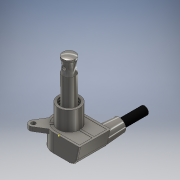
# Autodesk Inventor part: Peça 7
Saved by Autodesk Inventor 2016 (Build 200138000, 138)
## iProperties
Created: 2018-12-04
Part Number: Peça 7
Material: Generic
Document SubType Name: Sheet Metal
Designer: dqm_r
Density: 1 g/cm^3
Sheet Metal Rule: Default_mm
Appearance: Black
Author: dqm_r
Autodesk Inventor part; units mm, degrees
sketch "Sketch2" plane through (0, 0, 0) normal (0, 1, 0) x (-1, 0, 0)
  line L0 (10, 0) -> (-10, 0)
  line L1 (10, 0) -> (10, -9)
  line L2 (10, -9) -> (-5, -9)
  line L3 (-8.769781, -5.931826) -> (-10, 0)
  arc A0 (-8.769781, -5.931826) -> (-5, -9) centre (-5, -5.15) ccw
  line L4 (-10, 0) -> (-5, 0)
  point P0 (0, 0)
  point P1 (0, 0)
  dimension "d3" = 20
  dimension "d4" = 9
  dimension "d5" = 15
  dimension "d6" = 7.7
  dimension "d7" = 5
  constraints: 10 end point, 2 point on circle, 2 tangent, 1 centre point, 1 coincident, 1 horizontal, 1 midpoint, 1 perpendicular, 1 point on line, 1 vertical
  measures "d3" distance of L0.start L0.end
  measures "d4" distance of L0.start L1.end
  measures "d5" distance of L1.end L2.end
  measures "d6" diameter of A0
  measures "d7" distance of L0.end L4.end
extrude "Extrusion1" add sketch "Sketch2" along normal blind 15
sketch "Sketch3" plane through (-10, 0, 0) normal (0, 0, 1) x (1, 0, 0)
  arc A0 (7.5, 15) -> (0, 7.5) centre (7.5, 7.5) ccw
  line L0 (0, 7.5) -> (0, 15)
  line L1 (0, 15) -> (20, 15) projected
  line L2 (7.5, 15) -> (0, 15)
  line L3 (0, 15) -> (0, 7.5)
  line L4 (0, 0) -> (20, 0) projected
  line L5 (7.5, 0) -> (0, 0)
  point P0 (10, 0)
  constraints: 8 end point, 2 collinear, 2 point on circle, 1 centre point, 1 tangent
extrude "Extrusion2" cut sketch "Sketch3" against normal through all
ref_plane "Work Plane1" through (0, 7.5, 0) normal (0, 1, 0) x (1, 0, 0)
mirror "Mirror1" about plane through (0, 7.5, 0) normal (0, 1, 0) of "Extrusion2"
sketch "Sketch4" plane through (10, 0, 0) normal (0, 0, 1) x (1, 0, 0)
  line L0 (0, 0) -> (0, 15)
  line L1 (-19.947996, -2.700967) -> (-14.92788, 0.403846)
  circle A0 centre (-21, -1) radius 1
  line L2 (-12.5, 7.5) -> (-21, -1) construction
  line L3 (-12.5, 7.5) -> (-16.15365, 7.5) construction
  line L4 (-22.700211, 0.053225) -> (-19.594379, 5.066939)
  arc A1 (-19.594379, 5.066939) -> (-14.92788, 0.403846) centre (-12.5, 7.5) ccw
  arc A2 (-22.700211, 0.053225) -> (-19.947996, -2.700967) centre (-21, -1) ccw
  point P0 (-10, 0)
  point P1 (-18.400699, 2.870555)
  dimension "d51" = 45
  dimension "d55" = 2
  dimension "d57" = 4
  dimension "d125" = 8.5
  constraints: 8 end point, 4 point on circle, 3 centre point, 3 coincident, 2 tangent, 1 horizontal, 3 other
  measures "d51" angle of L3 L2
  measures "d55" diameter of A0
  measures "d57" diameter of A2
  measures "d125" horizontal distance of L2.end point (-12.5, 7.5)
extrude "Extrusion3" add sketch "Sketch4" against normal blind 2
sketch "Sketch5" plane through (10, 0, 0) normal (0, 0, 1) x (1, 0, 0)
  arc A0 (-12.5, 15) -> (-12.5, 0) centre (-12.5, 7.5) ccw projected
  circle A1 centre (-12.5, 7.5) radius 5.15
  circle A2 centre (-12.5, 7.5) radius 4
  point P0 (-10, 0)
  dimension "d22" = 10.3
  dimension "d23" = 8
  constraints: 2 centre point, 2 coincident
  measures "d22" diameter of A1
  measures "d23" diameter of A2
extrude "Extrusion4" add sketch "Sketch5" along normal blind 9
sketch "Sketch6" plane through (0, 15, 0) normal (0, 1, 0) x (1, 0, 0)
  arc A0 (8.769781, 5.931826) -> (5, 9) centre (5, 5.15) ccw
  circle A1 centre (5, 5.15) radius 3.75
  point P0 (0, 0)
  dimension "d26" = 7.5
  constraints: 1 centre point, 1 coincident
  measures "d26" diameter of A1
ref_plane "Work Plane2" through (0, 24, 0) normal (0, 1, 0) x (1, 0, 0)
sketch "Sketch7" plane through (0, 24, 0) normal (0, 1, 0) x (1, 0, 0)
  arc A0 (8.769781, 5.931826) -> (5, 9) centre (5, 5.15) ccw
  circle A1 centre (5, 5.15) radius 3.1
  point P0 (0, 0)
  dimension "d28" = 6.2
  constraints: 1 centre point, 1 coincident
  measures "d28" diameter of A1
loft "Loft1" add profiles "Sketch6", "Sketch7"
fillet "Fillet1" radius 0.5 7 edges at (7.4303, 15, -8.136) (1.25, 15, -9) (-10, 7.5, -9) (1.25, 0, -9) (7.4303, 0, -8.136) (9.3849, 0, -2.9659) (9.3849, 15, -2.9659)
sketch "Sketch8" plane through (5, 24, -5.15) normal (0, 1, 0) x (1, 0, 0)
  circle A0 centre (0, 0) radius 2.6
  point P0 (-5, -5.15)
  dimension "d34" = 5.2
  constraints: 1 centre point
  measures "d34" diameter of A0
hole "Hole1" at (5, 24, -5.15) direction (0, -1, 0) diameter 4.2 depth 20
sketch "Sketch9" plane through (-2.5, 0, 0) normal (0, 0, 1) x (1, 0, 0)
  line L0 (12.5, 0.5) -> (12.5, 14.5)
  line L1 (11.508493, 6.999) -> (11.508493, 0.999)
  line L2 (6.813999, 0.999) -> (11.508493, 0.999)
  line L3 (0.008493, 0.999) -> (6.813999, 0.999)
  line L4 (11.5, 8.000804) -> (11.5, 14.000804)
  line L5 (6.805507, 14.000804) -> (11.5, 14.000804)
  line L6 (0.445087, 13.990187) -> (6.805507, 14.000804)
  line L7 (11.508493, 6.999) -> (5.125573, 6.999)
  line L8 (11.5, 8.000804) -> (5.125592, 8.000804)
  line L9 (11.5, 7.5) -> (-9.863872, 7.5) construction
  arc A0 (0, 15) -> (-7.094379, 5.066939) centre (0, 7.5) ccw
  circle A1 centre (-8.5, -1) radius 1
  line L10 (0, 7.5) -> (-8.30271, 15.80271) construction
  arc A2 (0.445087, 13.990187) -> (-4.232874, 12.439981) centre (0, 7.5) ccw
  line L11 (0, 7.5) -> (-8.30271, -0.80271) construction
  line L12 (-3.97795, 10.770843) -> (-4.939981, 11.732874)
  line L13 (-4.232874, 12.439981) -> (-3.270843, 11.47795)
  line L14 (-4.056229, 10.849122) -> (-4.246481, 12.453588) construction
  line L15 (-4.953588, 11.746481) -> (-3.349122, 11.556229) construction
  line L16 (-5.125671, 7) -> (-6.486188, 7)
  line L17 (-6.505431, 8) -> (-5.125671, 8)
  line L18 (-3.97795, 4.229157) -> (-4.939981, 3.267126)
  line L19 (-4.232874, 2.560019) -> (-3.270843, 3.52205)
  arc A3 (-4.232874, 2.560019) -> (0.240072, 0.999) centre (0, 7.5) ccw
  arc A4 (-6.486188, 7) -> (-4.939981, 3.267126) centre (0, 7.5) ccw
  arc A5 (-4.939981, 11.732874) -> (-6.486188, 8) centre (0, 7.5) ccw
  arc A6 (-3.270843, 3.52205) -> (0, 2.35) centre (0, 7.5) ccw
  arc A7 (-5.125671, 7) -> (-3.97795, 4.229157) centre (0, 7.5) ccw
  arc A8 (-3.97795, 10.770843) -> (-5.125671, 8) centre (0, 7.5) ccw
  arc A9 (0.004263, 12.649998) -> (-3.270843, 11.47795) centre (0, 7.5) ccw
  arc A10 (-3.270843, 3.52205) -> (5.125573, 6.999) centre (0, 7.5) ccw
  arc A11 (5.125592, 8.000804) -> (-3.270843, 11.47795) centre (0, 7.5) ccw
  arc A12 (-3.97795, 10.770843) -> (-5.125671, 8) centre (0, 7.5) ccw
  arc A13 (-5.125671, 7) -> (-3.97795, 4.229157) centre (0, 7.5) ccw
  point P0 (2.5, 0)
  point P1 (-7.358951, 6.0523)
  point P2 (-4.151355, 11.651355)
  point P3 (-5.850772, 7.5)
  dimension "d48" = 6
  dimension "d50" = 45
  dimension "d126" = 0.501
  dimension "d127" = 0.5008
  dimension "d128" = 6
  constraints: 38 end point, 26 point on circle, 12 centre point, 5 point on line, 5 symmetric about line, 3 horizontal, 3 midpoint, 2 concentric, 2 parallel, 2 vertical, 1 coincident, 1 collinear, 1 perpendicular
  measures "d48" distance between parallel lines of L8 L5
  measures "d50" angle of L10 L9
  measures "d126" distance between parallel lines of L9 L7
  measures "d127" distance between parallel lines of L8 L9
  measures "d128" distance between parallel lines of L2 L7
extrude "Extrusion5" cut sketch "Sketch9" against normal blind 0.1 contours L1 L2 L3 A3 L19 A6 A10 L7 | L8 A11 A9 L13 A2 L6 L5 L4 | A8 L17 A5 L12 | A7 L18 A4 L16
thread "Thread1" size "M8x1.25" class "6H" standard "ANSI Metric M Profile" full length
sketch "Sketch10" plane through (-2.5, 0, -0.1) normal (0, 0, 1) x (1, 0, 0)
  point P0 (2.5, 0)
sketch "Sketch11" plane through (-2.5, 7.5, 0) normal (0, 0, 1) x (1, 0, 0)
  circle A0 centre (0, 0) radius 3
  point P0 (2.5, -7.5)
  dimension "d68" = 6
  constraints: 1 centre point
  measures "d68" diameter of A0
extrude "Extrusion6" add sketch "Sketch11" along normal blind 28
ref_plane "Work Plane4" through (0, 7.5, 0) normal (0, -1, 0) x (1, 0, 0)
sketch "Sketch16" plane through (0, 7.5, 0) normal (0, -1, 0) x (1, 0, 0)
  line L0 (0.5, 28) -> (-5.5, 28) projected
  line L1 (0.5, 28) -> (-2.5, 28)
  line L2 (-2.5, 28) -> (-2.5, 28.5)
  arc A0 (0.5, 28) -> (-2.5, 28.5) centre (-2.5, 19.25) ccw
  point P0 (0, 0)
  dimension "d85" = 0.5
  constraints: 5 end point, 2 point on circle, 1 centre point, 1 midpoint, 1 perpendicular
  measures "d85" distance of L2.end L1.end
revolve "Revolution1" add sketch "Sketch16" angle 360 about axis through (-2.5, 7.5, 28) along (0, 0, 1)
sketch "Sketch17" plane through (0, 7.5, 0) normal (0, -1, 0) x (1, 0, 0)
  point P0 (0, 0)
sketch "Sketch18" plane through (0, 7.5, 0) normal (0, -1, 0) x (1, 0, 0)
  line L0 (0.5, 28) -> (-5.5, 28)
  line L1 (-5.5, 28) -> (-5.5, 27)
  line L2 (-5.5, 0) -> (-5.5, 28)
  line L3 (-5.5, 27) -> (-5.5, 21)
  line L4 (-5.5, 24) -> (-5, 24)
  arc A0 (-5.5, 21) -> (-5.5, 27) centre (-14.25, 24) ccw
  line L5 (-5.5, 27) -> (-5.5, 21)
  line L6 (-2.5, 28) -> (-2.5, 20.788172) construction
  point P0 (0, 0)
  dimension "d87" = 1
  dimension "d89" = 0.5
  dimension "d108" = 6
  constraints: 10 end point, 3 point on circle, 2 midpoint, 2 point on line, 1 centre point, 1 collinear, 1 horizontal, 1 vertical
  measures "d87" distance of L0.end L1.end
  measures "d89" distance of L4.start L4.end
  measures "d108" distance of L3.end L1.end
revolve "Revolution2" cut sketch "Sketch18" angle 360 about axis through (-2.5, 7.5, 28) along (0, 0, -1)
ref_plane "Work Plane5" through (0, 2.5, 0) normal (0, -1, 0) x (1, 0, 0)
sketch "Sketch20" plane through (0, 2.5, 0) normal (0, -1, 0) x (1, 0, 0)
  line L0 (0.5, 27) -> (-5.5, 27) projected
  line L1 (-2.5, 27) -> (-2.5, 21) construction
  circle A0 centre (-2.5, 24) radius 1
  point P0 (0, 0)
  dimension "d100" = 2
  dimension "d109" = 6
  constraints: 2 end point, 2 midpoint, 1 centre point, 1 vertical
  measures "d100" diameter of A0
  measures "d109" distance of L1.start L1.end
hole "Hole3" at (-2.5, 2.5, 24) direction (0, 1, 0) diameter 2 end through all
sketch "Sketch21" plane through (5, 4, -5.15) normal (0, 1, 0) x (1, 0, 0)
  circle A0 centre (0, 0) radius 1.95
  point P0 (-5, -5.15)
  dimension "d110" = 3.9
  constraints: 1 centre point
  measures "d110" diameter of A0
extrude "Extrusion8" add sketch "Sketch21" along normal blind 32
sketch "Sketch22" plane through (5, 36, -5.15) normal (0, 1, 0) x (1, 0, 0)
  circle A0 centre (0, 0) radius 1.1
  point P0 (-5, -5.15)
  dimension "d113" = 2.2
  constraints: 1 centre point
  measures "d113" diameter of A0
hole "Hole4" at (5, 36, -5.15) direction (0, -1, 0) diameter 2 depth 7
thread "Thread2" size "M2x0.4" class "6H" standard "ANSI Metric M Profile" full length
equation "\"BendRadius\" = Thickness"
equation "\"BendReliefWidth\" = Thickness"
equation "\"BendReliefDepth\" = 0.5 * Thickness"
equation "\"CornerReliefSize\" = 4 * Thickness"
equation "\"MinimumRemnant\" = 2 * Thickness"
equation "\"TransitionRadius\" = BendRadius"
equation "\"JacobiRadiusSize\" = BendRadius"
equation "\"GapSize\" = Thickness"
equation "\"Thickness\" = 0.5"
body "Solid1"
